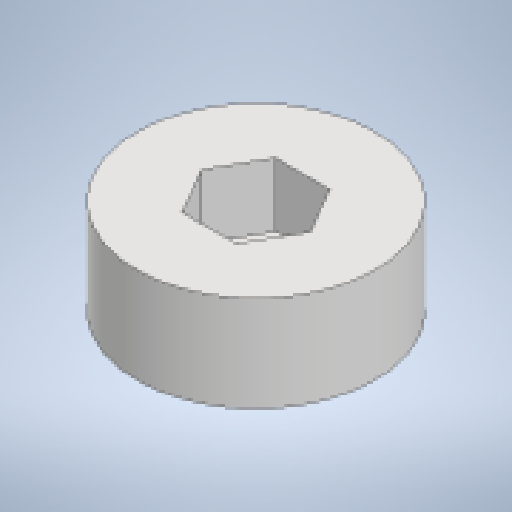
# Autodesk Inventor part: Cabeza_Tornillos
Saved by Autodesk Inventor 2024 (Build 280153000, 153)
## iProperties
Created: 2024-07-19
Part Number: Cabeza_Tornillos
Material: Genérico
Document SubType Name: Modeling
Designer: sergi
Density: 1 g/cm^3
Appearance: Valor por defecto
Author: sergi
Autodesk Inventor part; units mm, degrees
ref_plane "YZ Plane" through (0, 0, 0) normal (1, 0, 0) x (0, 1, 0)
ref_plane "XZ Plane" through (0, 0, 0) normal (0, 1, 0) x (-1, 0, 0)
ref_plane "XY Plane" through (0, 0, 0) normal (0, 0, 1) x (1, 0, 0)
sketch "Boceto1" plane through (0, 0, 0) normal (0, 1, 0) x (-1, 0, 0)
  line L0 (1.5588, -2.7) -> (-1.5588, -2.7)
  line L1 (-1.5588, -2.7) -> (-3.1177, 0)
  line L2 (-3.1177, 0) -> (-1.5588, 2.7)
  line L3 (-1.5588, 2.7) -> (1.5588, 2.7)
  line L4 (1.5588, 2.7) -> (3.1177, 0)
  line L5 (3.1177, 0) -> (1.5588, -2.7)
  line L6 (3.4064, 0) -> (1.7032, 2.95)
  line L7 (1.7032, 2.95) -> (-1.7032, 2.95)
  line L8 (-1.7032, 2.95) -> (-3.4064, 0)
  line L9 (-3.4064, 0) -> (-1.7032, -2.95)
  line L10 (-1.7032, -2.95) -> (1.7032, -2.95)
  line L11 (1.7032, -2.95) -> (3.4064, 0)
  circle A0 centre (0, 0) radius 7.5
  dimension "d0" = 5.4
  dimension "d1" = 0.25
  dimension "d2" = 15
  constraints: 24 end point, 2 coincident, 1 centre point, 1 horizontal, 18 other
  measures "d0" distance between parallel lines of L3 L0
  measures "d1" distance between parallel lines of L4 L6
  measures "d2" diameter of A0
extrude "Extrusión1" add sketch "Boceto1" along normal blind 6 contours L0 L1 L2 L3 L4 L5 | L11 L10 L9 L8 L7 L6 | A0
sketch "Boceto2" plane through (0, 6, 0) normal (0, 1, 0) x (1, 0, 0)
  line L0 (-3.1177, 0) -> (-1.5588, 2.7)
  line L1 (-1.5588, 2.7) -> (1.5588, 2.7)
  line L2 (1.5588, 2.7) -> (3.1177, 0)
  line L3 (3.1177, 0) -> (1.5588, -2.7)
  line L4 (1.5588, -2.7) -> (-1.5588, -2.7)
  line L5 (-1.5588, -2.7) -> (-3.1177, 0)
  line L6 (-3.4064, 0) -> (-1.7032, 2.95)
  line L7 (-1.7032, 2.95) -> (1.7032, 2.95)
  line L8 (1.7032, 2.95) -> (3.4064, 0)
  line L9 (3.4064, 0) -> (1.7032, -2.95)
  line L10 (1.7032, -2.95) -> (-1.7032, -2.95)
  line L11 (-1.7032, -2.95) -> (-3.4064, 0)
  point P0 (0, 0)
  point P1 (0, 0)
  dimension "d5" = 5.4
  dimension "d6" = 0.25
  constraints: 24 end point, 1 coincident, 1 horizontal, 18 other
  measures "d5" distance between parallel lines of L4 L1
  measures "d6" distance between parallel lines of L5 L11
extrude "Extrusión2" cut sketch "Boceto2" against normal blind 4 contours L0 L1 L2 L3 L4 L5 | L6 L7 L8 L9 L10 L11
sketch "Boceto3" plane through (0, 2, 0) normal (0, 1, 0) x (1, 0, 0)
  circle A0 centre (0, 0) radius 7.5 projected
  constraints: 1 coincident
hole "Agujero1" at (0, 2, 0) direction (0, -1, 0) diameter 3 end through all
